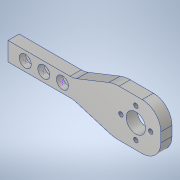
# Autodesk Inventor part: XmovementarmR
Saved by Autodesk Inventor 2020 (Build 240168000, 168)
## iProperties
Created: 2019-01-13
Part Number: XmovementarmR
Material: Aluminum 6061
Document SubType Name: Modeling
Designer: LillaHunden
Density: 2.7 g/cm^3
Appearance: Aluminum - Flat
Mass: 17.0465 g
Surface Area: 40.0048 cm^2
Volume: 6.31351 cm^3
Author: LillaHunden
Autodesk Inventor part; units mm, degrees
ref_plane "YZ Plane" through (0, 0, 0) normal (1, 0, 0) x (0, 1, 0)
ref_plane "XZ Plane" through (0, 0, 0) normal (0, 1, 0) x (-1, 0, 0)
ref_plane "XY Plane" through (0, 0, 0) normal (0, 0, 1) x (1, 0, 0)
sketch "Sketch1" plane through (0, 0, 0) normal (0, 0, 1) x (1, 0, 0)
  line L0 (86.8275, 18.5274) -> (61.537, 18.5274)
  line L1 (61.537, -6.6121) -> (86.8275, -6.6121)
  line L2 (86.8275, -6.6121) -> (86.8275, 18.5274)
  line L3 (6.25, 0) -> (40, 0) projected
  line L4 (40, 0) -> (40, 10) projected
  line L5 (4.75, 10) -> (40, 10) projected
  line L6 (61.537, 18.5274) -> (40, 10)
  circle A0 centre (34, 5) radius 2 projected
  line L7 (4.75, 10) -> (4.75, 1.5) projected
  circle A1 centre (14, 5) radius 1.5 projected
  circle A2 centre (34, 5) radius 1.5 projected
  circle A3 centre (24, 5) radius 1.5 projected
  line L8 (6.25, 0) -> (4.75, 1.5) projected
  line L9 (46, -2.9015) -> (46, 0) projected
  line L10 (46, 0) -> (40, 0)
  line L11 (40, 0) -> (61.537, -6.6121)
  circle A4 centre (73.4131, 5.9577) radius 2.5 construction
  line L12 (6.25, 0) -> (4.75, 0)
  line L13 (4.75, 0) -> (4.75, 1.5)
  point P0 (86.8275, 5.9577)
  constraints: 16 end point, 3 horizontal, 2 parallel, 2 vertical alignment, 1 horizontal alignment, 1 midpoint, 1 perpendicular
extrude "Extrusion1" add sketch "Sketch1" along normal blind 6 contours L2 L1 L11 L9 L10 L4 L6 L0 | L4 L3 L8 L7 L5 | L10 L9 L11 | L12 L13 L8 | A0 | A1 | A2 | A3
sketch "Sketch2" plane through (0, 0, 0) normal (0, 0, -1) x (-1, 0, 0)
  circle A0 centre (-73.4131, 5.9577) radius 2.5 construction
  circle A1 centre (-73.4131, 5.9577) radius 8 construction
  circle A2 centre (-73.4131, 5.9577) radius 8 construction
  circle A3 centre (-73.4131, 5.9577) radius 8 construction
  circle A4 centre (-73.4131, 5.9577) radius 8 construction
  point P0 (0, 0)
  point P1 (-81.4131, 5.9577)
  point P2 (-73.4131, -2.0423)
  point P3 (-65.4131, 5.9577)
  point P4 (-73.4131, 13.9577)
  dimension "d65" = 16
  dimension "d68" = 360
  constraints: 6 coincident, 2 horizontal alignment, 2 vertical alignment, 23 other
hole "Hole1" at (81.4131, 5.9577, 0) at (73.4131, -2.0423, 0) at (65.4131, 5.9577, 0) at (73.4131, 13.9577, 0) direction (0, 0, 1) diameter 2.459 depth 8.8 thread size "M3x0.5" class "6H" standard "ISO Metric profile"
sketch "Sketch3" plane through (0, 0, 6) normal (0, 0, 1) x (1, 0, 0)
  spline S0 degree 3 number of poles 994 construction
  circle A0 centre (73.4131, 5.9577) radius 2.5 construction
  circle A1 centre (73.4131, 5.9577) radius 5.2
  point P0 (0, 0)
  dimension "d56" = 10.4
  constraints: 1 centre point, 1 coincident
  measures "d56" diameter of A1
extrude "Extrusion2" cut sketch "Sketch3" against normal through all
sketch "Sketch4" plane through (0, 0, 6) normal (0, 0, 1) x (1, 0, 0)
  line L0 (4.75, 10) -> (4.75, 0) projected
  line L1 (4.75, 5.75) -> (48.7838, 5.75) construction
  point P0 (14.75, 5.75)
  point P1 (24.75, 5.75)
  point P2 (34.75, 5.75)
  point P3 (4.75, 1.5)
  dimension "d38" = 10
  dimension "d39" = 10
  dimension "d40" = 10
  constraints: 4 point on line, 2 end point, 1 horizontal
  measures "d38" distance of point (14.75, 5.75) L1.start
  measures "d39" distance of point (24.75, 5.75) point (14.75, 5.75)
  measures "d40" distance of point (34.75, 5.75) point (24.75, 5.75)
sketch "Sketch7" plane through (0, 0, 6) normal (0, 0, 1) x (1, 0, 0)
  point P0 (14, 5)
  point P1 (24, 5)
  point P2 (34, 5)
sketch "Sketch8" plane through (0, 0, 6) normal (0, 0, 1) x (1, 0, 0)
  point P0 (34, 5)
  point P1 (14, 5)
  point P2 (24, 5)
hole "Hole5" at (34, 5, 6) at (14, 5, 6) at (24, 5, 6) direction (0, 0, -1) diameter 3.4 depth 6 counterbore diameter 6.5 counterbore depth 3.4
fillet "Fillet4" radius 10 2 edges at (86.8275, 18.5274, 3) (86.8275, -6.6121, 3)
fillet "Fillet5" radius 15 2 edges at (61.537, 18.5274, 3) (61.537, -6.6121, 3)
fillet "Fillet6" radius 10 2 edges at (40, 10, 3) (40, 0, 3)
equation "\"d13\" = d11"
equation "\"d11\" = 14"
body "Solid1"
